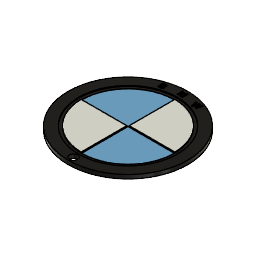
BMW_Logo_Keychain (Autodesk Fusion 360 design; units mm, degrees)
part number: 2026-08-15-03-22-54-718
Autodesk Fusion 360 part; units mm, degrees
sketch "Logo_Profile" plane through (0, 0, 0) normal (0, 0, 1) x (1, 0, 0)
  circle A0 centre (0, 0) radius 30
  circle A1 centre (0, 0) radius 24
  circle A2 centre (0, 0) radius 17
  line L0 (-17, 0) -> (17, 0) construction
  line L1 (0, -17) -> (0, 17) construction
  dimension "d1" = 60
  dimension "d2" = 48
  dimension "d3" = 34
  dimension "d4" = 34
  constraint coincident A0.centre A1.centre
  constraint concentric A0 A1
  constraint concentric A1 A2
  constraint horizontal L0
  constraint vertical L1
  constraint midpoint A0.centre L0
  constraint midpoint A0.centre L1
  constraint equal L0 L1
  measures "d1" diameter of A0
  measures "d2" diameter of A1
  measures "d3" diameter of A2
  measures "d4" horizontal distance of L0.start L0.end
sketch "Keychain_Hole" plane through (0, 0, 0) normal (0, 0, 1) x (1, 0, 0)
  circle A0 centre (0, -27.375) radius 2
  line L0 (0, 0) -> (0, -27.375) construction
  dimension "d5" = 4
  dimension "d6" = -27.375
  constraint vertical L0
  constraint coincident L0.start origin
  constraint coincident A0.centre L0.end
  measures "d5" diameter of A0
  measures "d6" vertical distance of L0.start A0.centre
extrude "Main_Extrude" add sketch "Logo_Profile" along normal blind 2 contours A0 | A1 | A2
extrude "Keychain_Hole_Cut" cut sketch "Keychain_Hole" along normal through all
sketch "Inner_Ring" plane through (0, 0, 2) normal (0, 0, 1) x (1, 0, 0)
  circle A0 centre (0, -27.375) radius 2
  circle A1 centre (0, 0) radius 30
  circle A2 centre (0, 0) radius 24.75
  circle A3 centre (0, 0) radius 23.25
  dimension "d20" = 49.5
  dimension "d21" = 46.5
  constraint concentric A2 A3
  constraint coincident A1.centre A2.centre
  measures "d20" diameter of A2
  measures "d21" diameter of A3
extrude "Inner_Ring_Cut" cut sketch "Inner_Ring" against normal blind 0.4 contours A2
sketch "BMW_Text" plane through (0, 0, 2) normal (0, 0, 1) x (1, 0, 0)
  circle A0 centre (0, 0) radius 30
  circle A1 centre (0, -27.375) radius 2
  circle A2 centre (0, 0) radius 24.75
  line L0 (-12.5, 22.51) -> (-4.5, 22.51) construction
  line L1 (-4.5, 22.51) -> (-4.5, 29.51) construction
  line L2 (-4.5, 29.51) -> (-12.5, 29.51) construction
  line L3 (-12.5, 29.51) -> (-12.5, 22.51) construction
  line L4 (-4, 23.875) -> (4, 23.875) construction
  line L5 (4, 23.875) -> (4, 30.875) construction
  line L6 (4, 30.875) -> (-4, 30.875) construction
  line L7 (-4, 30.875) -> (-4, 23.875) construction
  line L8 (4.5, 22.51) -> (12.5, 22.51) construction
  line L9 (12.5, 22.51) -> (12.5, 29.51) construction
  line L10 (12.5, 29.51) -> (4.5, 29.51) construction
  line L11 (4.5, 29.51) -> (4.5, 22.51) construction
  dimension "d39" = 2.8
  dimension "d41" = 2.8
  dimension "d43" = 2.8
  text T0 "B" font "Arial" height 2.8 bold align centre middle in box 8 x 7 at (-12.5, 22.51) x (1, 0) y (0, 1) spacing 1
  text T1 "M" font "Arial" height 2.8 bold align centre middle in box 8 x 7 at (-4, 23.875) x (1, 0) y (0, 1) spacing 1
  text T2 "W" font "Arial" height 2.8 bold align centre middle in box 8 x 7 at (4.5, 22.51) x (1, 0) y (0, 1) spacing 1
extrude "BMW_Text_Engraving" cut sketch "BMW_Text" against normal blind 0.35 text T0 T1 T2
sketch "Quadrant_Division" plane through (0, 0, 2) normal (0, 0, 1) x (1, 0, 0)
  circle A0 centre (0, 0) radius 23.25
  circle A1 centre (0, 0) radius 23.25
  line L0 (-23.25, 0) -> (23.25, 0)
  line L1 (0, -23.25) -> (0, 23.25)
  dimension "d47" = 46.5
  constraint coincident A0.centre A1.centre
  constraint horizontal L0
  constraint vertical L1
  constraint midpoint A0.centre L0
  constraint midpoint A0.centre L1
  constraint coincident A1 L0.start
  constraint coincident A1 L1.start
  measures "d47" diameter of A1
extrude "Quadrant_Recess" cut sketch "Quadrant_Division" against normal blind 0.35 contours A0 A1 L0 L1 | A0 A1 L0 L1 picked at (15.4211, -1.1029) picked at (-15.4211, 1.1029)
ref_plane "WorkPlane1" through (0, 0, 2) normal (0, 0, 1) x (1, 0, 0)
sketch "Division_Groove" plane through (0, 0, 2) normal (0, 0, 1) x (1, 0, 0)
  line L0 (-23.25, -0.3) -> (23.25, -0.3)
  line L1 (23.25, -0.3) -> (23.25, 0.3)
  line L2 (23.25, 0.3) -> (-23.25, 0.3)
  line L3 (-23.25, 0.3) -> (-23.25, -0.3)
  line L4 (-23.25, -0.3) -> (23.25, 0.3) construction
  line L5 (-0.3, -23.25) -> (0.3, -23.25)
  line L6 (0.3, -23.25) -> (0.3, 23.25)
  line L7 (0.3, 23.25) -> (-0.3, 23.25)
  line L8 (-0.3, 23.25) -> (-0.3, -23.25)
  line L9 (-0.3, -23.25) -> (0.3, 23.25) construction
  dimension "d58" = 46.5
  dimension "d59" = 0.6
  dimension "d60" = 46.5
  dimension "d61" = 0.6
  constraint horizontal L0
  constraint horizontal L2
  constraint vertical L1
  constraint vertical L3
  constraint midpoint origin L4
  constraint horizontal L5
  constraint horizontal L7
  constraint vertical L6
  constraint vertical L8
  constraint midpoint origin L9
  measures "d58" horizontal distance of L0.start L0.end
  measures "d59" vertical distance of L0.end L1.end
  measures "d60" vertical distance of L5.end L6.end
  measures "d61" horizontal distance of L5.start L5.end
extrude "Division_Groove_Cut" cut sketch "Division_Groove" against normal blind 0.3
equation "d22 = -( 0.40 mm )"
equation "d40 = 'B'"
equation "d42 = 'M'"
equation "d44 = 'W'"
equation "d45 = -( 0.35 mm )"
equation "d50 = -( 0.35 mm )"
equation "d62 = -( 0.30 mm )"
named bodies: "BMW_Logo_Keychain_Body"
